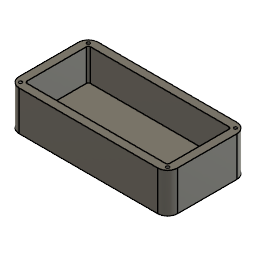
Box_Assembly_with screws (Autodesk Fusion 360 archive; units mm, degrees)
design "Box"
part number: 2026-05-18-14-11-44-767
Autodesk Fusion 360 part; units mm, degrees
note: some values were not read from the file. Chosen so that the rebuilt part matches the saved one: which face or edge a step refers to.
sketch "Sketch1" plane through (0, 0, 0) normal (0, 1, 0) x (1, 0, 0)
  line L0 (35, 20) -> (-35, 20)
  line L1 (-40, 15) -> (-40, -15)
  line L2 (-35, -20) -> (35, -20)
  line L3 (40, -15) -> (40, 15)
  line L4 (40, 20) -> (-40, -20) construction
  line L5 (-40, 20) -> (40, -20) construction
  arc A0 (-35, 20) -> (-40, 15) centre (-35, 15) ccw
  arc A1 (40, 15) -> (35, 20) centre (35, 15) ccw
  arc A2 (35, -20) -> (40, -15) centre (35, -15) ccw
  arc A3 (-40, -15) -> (-35, -20) centre (-35, -15) ccw
  line L6 (-36, 15) -> (-36, -15)
  arc A4 (-36, -15) -> (-35, -16) centre (-35, -15) ccw
  line L7 (-35, -16) -> (35, -16)
  arc A5 (35, -16) -> (36, -15) centre (35, -15) ccw
  line L8 (36, -15) -> (36, 15)
  arc A6 (36, 15) -> (35, 16) centre (35, 15) ccw
  line L9 (35, 16) -> (-35, 16)
  arc A7 (-35, 16) -> (-36, 15) centre (-35, 15) ccw
  dimension "d1" = 80
  dimension "d2" = 40
  dimension "d3" = 5
  dimension "d4" = -4
  constraint horizontal L0
  constraint perpendicular L0 L1
  constraint parallel L0 L2
  constraint parallel L1 L3
  constraint coincident L4 origin
  constraint coincident L5 origin
  constraint coincident L5.start L1
  constraint coincident L5.start L0
  constraint tangent L1 A0
  constraint tangent L0 A0
  constraint coincident L4.start L0
  constraint coincident L4.start L3
  constraint tangent L0 A1
  constraint tangent L3 A1
  constraint equal A0 A1
  constraint coincident L5.end L3
  constraint coincident L5.end L2
  constraint tangent L3 A2
  constraint tangent L2 A2
  constraint equal A0 A2
  constraint coincident L4.end L2
  constraint coincident L4.end L1
  constraint tangent L2 A3
  constraint tangent L1 A3
  constraint equal A0 A3
  measures "d1" distance of L4.end L5.end
  measures "d2" distance of L5.start L4.end
  measures "d3" radius of A0
extrude "Extrude1" add sketch "Sketch1" along normal blind 4 contours L6 A4 L7 A5 L8 A6 L9 A7
extrude "Extrude2" add sketch "Sketch1" along normal blind 20
sketch "Sketch2" plane through (0, 20, 0) normal (0, 1, 0) x (-1, 0, 0)
  arc A0 (35, -16) -> (36, -15) centre (35, -15) ccw
  line L0 (35, -16) -> (-35, -16)
  arc A1 (-36, -15) -> (-35, -16) centre (-35, -15) ccw
  line L1 (-36, -15) -> (-36, 15)
  arc A2 (-35, 16) -> (-36, 15) centre (-35, 15) ccw
  line L2 (-35, 16) -> (35, 16)
  arc A3 (36, 15) -> (35, 16) centre (35, 15) ccw
  line L3 (36, 15) -> (36, -15)
  arc A4 (40, 15) -> (35, 20) centre (35, 15) ccw
  line L4 (35, 20) -> (-35, 20)
  arc A5 (-35, 20) -> (-40, 15) centre (-35, 15) ccw
  line L5 (-40, 15) -> (-40, -15)
  arc A6 (-40, -15) -> (-35, -20) centre (-35, -15) ccw
  line L6 (-35, -20) -> (35, -20)
  arc A7 (35, -20) -> (40, -15) centre (35, -15) ccw
  line L7 (40, -15) -> (40, 15)
  line L8 (37.12, 17.12) -> (-37.12, 17.12)
  line L9 (-37.12, 17.12) -> (-37.12, -17.12)
  line L10 (-37.12, -17.12) -> (37.12, -17.12)
  line L11 (37.12, -17.12) -> (37.12, 17.12)
  line L12 (37.12, 17.12) -> (-37.12, -17.12) construction
  line L13 (-37.12, 17.12) -> (37.12, -17.12) construction
  dimension "d9" = 74.24
  dimension "d10" = 34.24
  constraint horizontal L8
  constraint perpendicular L8 L9
  constraint parallel L8 L10
  constraint parallel L9 L11
  constraint coincident L12 origin
  constraint coincident L13 origin
  measures "d9" distance of L9.end L10.end
  measures "d10" distance of L8.end L9.end
hole "Hole1" at (37.12, 20, 17.12) at (-37.12, 20, 17.12) at (-37.12, 20, -17.12) at (37.12, 20, -17.12) direction (0, -1, 0) diameter 1.471 depth 11 tip angle 118
thread "Thread1" "ISO Metric profile 1.8 M1.8x0.35 M1.8x0.35 6H" major diameter 1.8678 minor diameter 1.4711 pitch 0.35 angle 60 resizes the face on face at (-37.7172, 16.3333, 17.5493) on face at (36.5228, 16.3333, 17.5493) on face at (-37.7172, 16.3333, -16.6907) on face at (36.5228, 16.3333, -16.6907)
